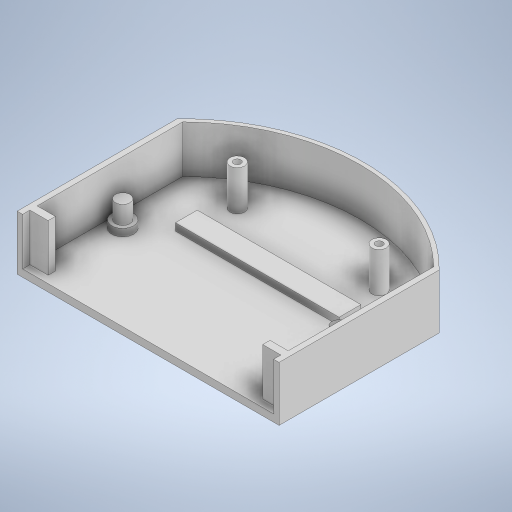
# Autodesk Inventor part: Spiel
Saved by Autodesk Inventor 2024 (Build 280153000, 153)
## iProperties
Created: 2024-01-17
Part Number: Spiel
Material: Generisch
Document SubType Name: Modeling
Designer: User
Density: 1 g/cm^3
Appearance: Vorgabe
Author: User
Autodesk Inventor part; units mm, degrees
ref_plane "YZ Plane" through (0, 0, 0) normal (1, 0, 0) x (0, 1, 0)
ref_plane "XZ Plane" through (0, 0, 0) normal (0, 1, 0) x (-1, 0, 0)
ref_plane "XY Plane" through (0, 0, 0) normal (0, 0, 1) x (1, 0, 0)
sketch "Skizze1" plane through (0, 0, 0) normal (0, 0, 1) x (1, 0, 0)
  line L0 (-20.1131, -4) -> (51.8869, -4)
  line L1 (51.8869, -4) -> (51.8869, 40)
  line L2 (51.8869, 40) -> (-20.1131, 40)
  line L3 (-20.1131, 40) -> (-20.1131, -4)
  arc A0 (51.8869, 40) -> (-20.1131, 40) centre (15.8869, 5.3013) ccw
  line L4 (50.3869, -4) -> (50.3869, 40)
  line L5 (-18.6131, 40) -> (-18.6131, -4)
  arc A1 (50.3869, 40) -> (-18.6131, 40) centre (15.8869, 5.2581) ccw
  point P0 (0, 0)
  dimension "d0" = 72
  dimension "d1" = 44
  dimension "d2" = 50
  dimension "d3" = 1.5
  dimension "d4" = 1.5
  constraints: 12 end point, 4 point on circle, 4 point on line, 3 parallel, 2 centre point, 1 horizontal, 1 perpendicular
  measures "d0" distance of L2.end L1.end
  measures "d1" distance of L1.end L0.end
  measures "d2" radius of A0
  measures "d3" distance between parallel lines of L1 L4
  measures "d4" distance between parallel lines of L3 L5
extrude "Extrusion1" add sketch "Skizze1" along normal blind 2 contours L5 L2 L4 L0 | A1 L2
extrude "Extrusion2" add sketch "Skizze1" along normal blind 15 contours L3 L2 L5 L0 | A0 L2 A1 | L4 L2 L1 L0
sketch "Skizze2" plane through (0, 0, 2) normal (0, 0, 1) x (1, 0, 0)
  circle A0 centre (-14.6131, 19.5) radius 3
  circle A1 centre (-14.6131, 19.5) radius 2
  circle A2 centre (45.3869, 19) radius 3
  circle A3 centre (45.3869, 19) radius 2
  line L0 (50.3869, 40) -> (50.3869, -4) projected
  line L1 (-18.6131, -4) -> (-18.6131, 40) projected
  circle A4 centre (-3.6131, 40) radius 2
  circle A5 centre (35.3869, 40) radius 2
  circle A6 centre (35.3869, 40) radius 1
  circle A7 centre (-3.6131, 40) radius 1
  line L2 (-6.6131, 32) -> (38.3869, 32)
  line L3 (38.3869, 32) -> (38.3869, 26)
  line L4 (38.3869, 26) -> (-6.6131, 26)
  line L5 (-6.6131, 26) -> (-6.6131, 32)
  line L6 (50.3869, -4) -> (43.3869, -4)
  line L7 (-18.6131, 0) -> (-13.6131, 0)
  line L8 (-13.6131, 0) -> (-13.6131, -2)
  line L9 (-13.6131, -2) -> (-18.6131, -2)
  line L10 (-18.6131, -2) -> (-18.6131, 0)
  line L11 (45.3869, 0) -> (50.3869, 0)
  line L12 (50.3869, 0) -> (50.3869, -2)
  line L13 (50.3869, -2) -> (45.3869, -2)
  line L14 (45.3869, -2) -> (45.3869, 0)
  line L15 (-18.6131, -4) -> (50.3869, -4) projected
  point P0 (0, 0)
  point P1 (15.8869, 26)
  point P2 (15.8869, 32)
  point P3 (-6.6131, 29)
  point P4 (38.3869, 29)
  point P5 (45.3869, -1)
  point P6 (-13.6131, -1)
  dimension "d9" = 6
  dimension "d10" = 4
  dimension "d11" = 6
  dimension "d12" = 4
  dimension "d13" = 5
  dimension "d14" = 4
  dimension "d21" = 4
  dimension "d22" = 4
  dimension "d23" = 2
  dimension "d24" = 2
  dimension "d27" = 15
  dimension "d28" = 15
  dimension "d29" = 60
  dimension "d30" = 6
  dimension "d31" = 45
  dimension "d32" = 12
  dimension "d33" = 12
  dimension "d40" = 5
  dimension "d41" = 2
  dimension "d43" = 5
  dimension "d44" = 2
  dimension "d45" = 2
  dimension "d46" = 59
  dimension "d47" = 23.5
  dimension "d48" = 23
  dimension "d49" = 44
  dimension "d50" = 44
  dimension "d51" = 30
  constraints: 26 end point, 8 centre point, 6 midpoint, 6 parallel, 4 coincident, 4 horizontal, 3 perpendicular, 2 point on line
  measures "d9" diameter of A0
  measures "d10" diameter of A1
  measures "d11" diameter of A2
  measures "d12" diameter of A3
  measures "d13" distance from line of L0 A2.centre
  measures "d14" distance from line of L1 A0.centre
  measures "d21" diameter of A4
  measures "d22" diameter of A5
  measures "d23" diameter of A6
  measures "d24" diameter of A7
  measures "d27" distance from line of L1 A4.centre
  measures "d28" distance from line of L0 A5.centre
  measures "d29" horizontal distance of A2.centre A0.centre
  measures "d30" distance of point (15.887, 26) point (15.887, 32)
  measures "d31" distance of L2.start L2.end
  measures "d32" distance from line of L1 point (-6.613, 29)
  measures "d33" distance from line of L0 point (38.387, 29)
  measures "d40" distance of L8.end L9.end
  measures "d41" distance of L7.end L8.end
  measures "d43" distance of L12.end L13.end
  measures "d44" distance between parallel lines of L13 L11
  measures "d45" distance between parallel lines of L6 L13
  measures "d46" distance of point (45.387, -1) point (-13.613, -1)
  measures "d47" distance from line of L15 A0.centre
  measures "d48" distance from line of L15 A2.centre
  measures "d49" distance from line of L15 A5.centre
  measures "d50" distance from line of L15 A4.centre
  measures "d51" distance between parallel lines of L15 L4
extrude "Extrusion3" add sketch "Skizze2" along normal blind 2 contours A0 | A2 | L2 L3 L4 L5
extrude "Extrusion4" add sketch "Skizze2" along normal blind 7 contours A1 | A3
extrude "Extrusion5" add sketch "Skizze2" along normal blind 11 contours A4 | A5
extrude "Extrusion6" add sketch "Skizze2" along normal up to surface (13 mm away) contours L0 L13 L14 L11 | L1 L7 L8 L9
